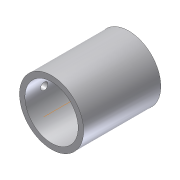
# Autodesk Inventor part: FE-00013-02
Saved by Autodesk Inventor 2012 (Build 160160000, 160)
## iProperties
Created: 2008-05-28
Part Number: FE-00013-02
Description: Bottom Coupling
Document SubType Name: Modeling
Designer: narosenberg
Density: 1 g/cm^3
Mass: 21.7902 g
Surface Area: 132.205 cm^2
Volume: 21.7902 cm^3
Material: Default
Author: narosenberg
Autodesk Inventor part; units mm, degrees
ref_plane "XZ Plane" through (0, 0, 0) normal (0, 1, 0) x (-1, 0, 0)
ref_plane "XY Plane" through (0, 0, 0) normal (0, 0, 1) x (1, 0, 0)
sketch "Sketch1" plane through (0, 0, 0) normal (0, 0, 1) x (1, 0, 0)
  circle A0 centre (-7.7519, 8.9922) radius 21.082
  circle A1 centre (-7.7519, 8.9922) radius 17.526
  dimension "d0" = 42.164
  dimension "d1" = 35.052
  constraints: 2 centre point, 1 coincident
  measures "d0" diameter of A0
  measures "d1" diameter of A1
extrude "Extrusion1" add sketch "Sketch1" along normal blind 50.8
ref_plane "Work Plane1" through (-28.8339, 8.9922, 0) normal (1, 0, 0) x (0, 1, 0)
sketch "Sketch2" plane through (-28.8339, 8.9922, 0) normal (1, 0, 0) x (0, 1, 0)
  line L0 (0, -10.16) -> (0, 60.96) projected
  line L1 (-17.526, 50.8) -> (17.526, 50.8) projected
  line L2 (-21.082, 50.8) -> (21.082, 50.8) projected
  line L3 (-21.082, 50.8) -> (21.082, 50.8) projected
  line L4 (-21.082, 0) -> (21.082, 0) projected
  line L5 (0, 0) -> (0, 50.8) projected
  line L6 (21.082, 0) -> (21.082, 50.8) projected
  line L7 (-21.082, 0) -> (-21.082, 50.8) projected
  circle A0 centre (0, 12.7) radius 2.3813
  circle A1 centre (0, 38.1) radius 2.3813
  dimension "d4" = 12.7
  dimension "d5" = 12.7
  dimension "d6" = 4.7625
  dimension "d7" = 4.7625
  constraints: 2 centre point, 2 point on line
  measures "d4" distance from line of A0.centre L4
  measures "d5" distance from line of A1.centre L1
  measures "d6" diameter of A1
  measures "d7" diameter of A0
extrude "Extrusion2" cut sketch "Sketch2" along normal up to next contours A0 L0 | L0 A0 | A1 L0 | L0 A1
body "Solid1"
